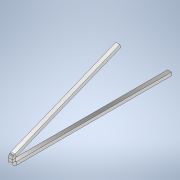
# Autodesk Inventor part: RJ45 Odd Pins
Saved by Autodesk Inventor 2020.1 (Build 241239000, 239)
## iProperties
Created: 2019-12-05
Part Number: RJ45 Odd Pins
Material: Nickel-Copper Alloy 400
Document SubType Name: Sheet Metal
Designer: S. Lee
Mass: 0.0429968 g
Surface Area: 0.498771 cm^2
Volume: 0.0048694 cm^3
Density: 8.83 g/cm^3
Sheet Metal Rule: Nickel Copper Alloy
Appearance: Chrome - Polished
Author: S. Lee
Autodesk Inventor part; units mm, degrees
ref_plane "YZ Plane" through (0, 0, 0) normal (1, 0, 0) x (0, 1, 0)
ref_plane "XZ Plane" through (0, 0, 0) normal (0, 1, 0) x (-1, 0, 0)
ref_plane "XY Plane" through (0, 0, 0) normal (0, 0, 1) x (1, 0, 0)
sketch "Sketch1" plane through (0, 0, 0) normal (0, 1, 0) x (-1, 0, 0)
  line L0 (0.224, 8.675) -> (-0.224, 8.675)
  line L1 (-0.224, 8.675) -> (-0.224, -8.675)
  line L2 (-0.224, -8.675) -> (0.224, -8.675)
  line L3 (0.224, -8.675) -> (0.224, 8.675)
  line L4 (0.224, 8.675) -> (-0.224, -8.675) construction
  line L5 (-0.224, 8.675) -> (0.224, -8.675) construction
  point P0 (0, 0)
  dimension "d0" = 0.448
  dimension "d1" = 17.35
  measures "d0" distance of L2.end L1.end
  measures "d1" distance of L0.end L1.end
extrude "Plate1" add sketch "Sketch1" along normal blind 0.35
sketch "Sketch2" plane through (0.224, 0.45, 8.775) normal (0, 0, 1) x (1, 0, 0)
  line L0 (-0.448, 0) -> (0, 0)
  line L1 (0, 0) -> (0, 0.3)
  line L2 (0, 0.3) -> (-0.448, 0.3)
  line L3 (-0.448, 0.3) -> (-0.448, 0)
  constraints: 6 end point, 1 horizontal, 1 perpendicular, 1 vertical
edge flange "Flange1" height 0.75 angle 90 thickness 0.35 bend radius 0.1 thickness toward (0, 0, 1) relief tear relief width 0.35 relief depth 0.175 edges at (0, 0.35, 8.675) wall of the first edge with corners at (-0.224, 0.45, 8.775) (0.224, 0.45, 8.775) (0.224, 0.75, 8.775) (-0.224, 0.75, 8.775)
bend "Bend1"
corner "Corner1"
sketch "Sketch3" plane through (0.224, 0.8427, 8.7125) normal (0, 0.9271839, 0.3746066) x (-1, 0, 0)
  line L0 (0.448, 0) -> (0, 0)
  line L1 (0, 0) -> (0, -12.6465)
  line L2 (0, -12.6465) -> (0.448, -12.6465)
  line L3 (0.448, -12.6465) -> (0.448, 0)
  constraints: 6 end point, 1 horizontal, 1 perpendicular, 1 vertical
edge flange "Flange2" height 12.95 angle 68 thickness 0.35 bend radius 0.1 thickness toward (0, 0.9271839, 0.3746066) relief tear relief width 0.35 relief depth 0.175 edges at (0, 0.75, 8.775) wall of the first edge with corners at (-0.224, 0.8427, 8.7125) (0.224, 0.8427, 8.7125) (0.224, 5.5802, -3.0131) (-0.224, 5.5802, -3.0131)
bend "Bend2"
corner "Corner2"
equation "\"d2\" = Thickness"
equation "\"d3\" = BendReliefWidth"
equation "\"d4\" = BendReliefDepth"
equation "\"d5\" = MinimumRemnant"
equation "\"d6\" = TransitionRadius"
equation "\"d9\" = BendRadius"
equation "\"d10\" = CornerReliefSize"
equation "\"d11\" = GapSize"
equation "\"d12\" = JacobiRadiusSize"
equation "\"d13\" = BendReliefWidth"
equation "\"d14\" = BendReliefDepth"
equation "\"d15\" = MinimumRemnant"
equation "\"d16\" = TransitionRadius"
equation "\"d19\" = BendRadius"
equation "\"d20\" = CornerReliefSize"
equation "\"d21\" = GapSize"
equation "\"d22\" = JacobiRadiusSize"
equation "\"BendReliefWidth\" = Thickness"
equation "\"BendReliefDepth\" = 0.5 * Thickness"
equation "\"CornerReliefSize\" = 4 * Thickness"
equation "\"MinimumRemnant\" = 2 * Thickness"
equation "\"TransitionRadius\" = BendRadius"
equation "\"JacobiRadiusSize\" = BendRadius"
equation "\"GapSize\" = Thickness"
equation "\"Thickness\" = 0.35"
equation "\"BendRadius\" = 0.1"
body "Solid1"
